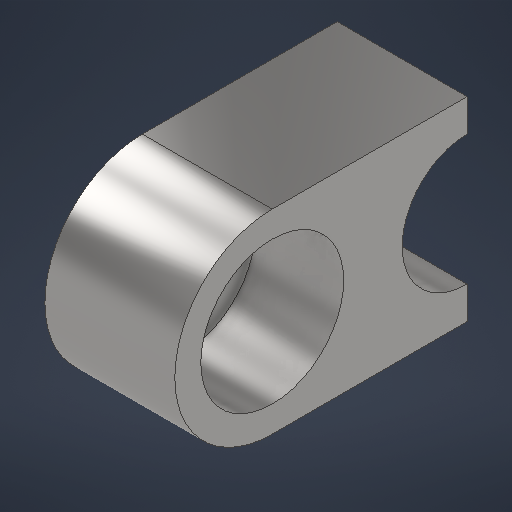
# Autodesk Inventor part: Part7
Saved by Autodesk Inventor 2026 (Build 300175000, 175)
## iProperties
Created: 2026-03-22
Part Number: Part7
Material: Generic
Document SubType Name: Modeling
Designer: Mlinč
Density: 1 g/cm^3
Appearance: Default
Author: Mlinč
Autodesk Inventor part; units mm, degrees
ref_plane "YZ Plane" through (0, 0, 0) normal (1, 0, 0) x (0, 1, 0)
ref_plane "XZ Plane" through (0, 0, 0) normal (0, 1, 0) x (-1, 0, 0)
ref_plane "XY Plane" through (0, 0, 0) normal (0, 0, 1) x (1, 0, 0)
sketch "Sketch1" plane through (0, 0, 0) normal (1, 0, 0) x (0, 1, 0)
  line L0 (0, 0) -> (0, -30) construction
  line L1 (-7.5, 0) -> (-7.5, -30)
  line L2 (7.5, -30) -> (7.5, 0)
  arc A0 (7.5, 0) -> (-7.5, 0) centre (0, 0) ccw
  arc A1 (-7.5, -30) -> (7.5, -30) centre (0, -30) ccw
  point P0 (0, -15)
  dimension "d0" = 7.5
  dimension "d1" = 30
  constraints: 8 end point, 4 point on circle, 4 tangent, 2 centre point, 1 midpoint, 1 parallel, 1 vertical
  measures "d0" radius of A0
  measures "d1" distance of L2.start L2.end
extrude "Extrusion1" add sketch "Sketch1" against normal blind 10
sketch "Sketch2" plane through (0, 0, 0) normal (1, 0, 0) x (0, 0, -1)
  line L0 (37.5, -7.5) -> (15, -7.5)
  line L1 (15, -7.5) -> (15, 7.5)
  line L2 (15, 7.5) -> (37.5, 7.5)
  line L3 (37.5, 7.5) -> (37.5, -7.5)
  arc A0 (30, -7.5) -> (30, 7.5) centre (30, 0) ccw projected
  line L4 (0, -7.5) -> (30, -7.5) projected
  line L5 (30, 7.5) -> (0, 7.5) projected
  point P0 (0, 0)
  point P1 (37.5, 0)
  point P2 (26.25, -7.5)
  point P3 (26.25, 7.5)
  point P4 (30, 7.5)
  point P5 (30, -7.5)
  dimension "d4" = 22.5
  constraints: 8 end point, 3 midpoint, 2 parallel, 2 point on line, 1 horizontal, 1 perpendicular, 1 point on circle
  measures "d4" distance between parallel lines of L3 L1
extrude "Extrusion2" cut sketch "Sketch2" against normal blind 10 contours L0 L1 L2 A0
sketch "Sketch3" plane through (0, 0, 0) normal (1, 0, 0) x (0, 0, -1)
  circle A0 centre (0, 0) radius 3.3
  line L0 (15, -7.5) -> (15, 7.5) projected
  point P0 (0, 0)
  dimension "d7" = 6.6
  constraints: 1 centre point
  measures "d7" diameter of A0
extrude "Extrusion3" cut sketch "Sketch3" against normal blind 10
sketch "Sketch4" plane through (0, 0, 0) normal (1, 0, 0) x (0, 0, -1)
  circle A0 centre (0, 0) radius 5.5
  dimension "d11" = 11
  constraints: 1 centre point, 1 coincident
  measures "d11" diameter of A0
extrude "Extrusion4" cut sketch "Sketch4" against normal blind 6.8
sketch "Sketch5" plane through (0, 0, 0) normal (1, 0, 0) x (0, 0, -1)
  line L0 (15, -7.5) -> (15, 7.5) projected
  circle A0 centre (15, 0) radius 5
  point P0 (0, 0)
  point P1 (15, 5)
  point P2 (15, -5)
  dimension "d14" = 10
  constraints: 1 centre point, 1 midpoint
  measures "d14" diameter of A0
extrude "Extrusion5" cut sketch "Sketch5" against normal through all contours A0 L0 picked at (13.3455, -0.2009)
body "Solid1"
